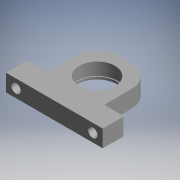
# Autodesk Inventor part: C-BGHKA6902ZZ-30_b_b
Saved by Autodesk Inventor 2017.3 (Build 213256000, 256)
## iProperties
Part Number: C-BGHKA6902ZZ-30_b_b
Material: Generic
Catalog Web Link: www.cadenas.de
Description: C-BGHKA_body-C-VALUE Medium Accuracy Bearings with Housings - T-Shaped
Vendor: MISUMI
Document SubType Name: Modeling
Designer: partserver
Manufacturer: MISUMI
Mass: 19.5015 g
Surface Area: 79.3385 cm^2
Volume: 19.5015 cm^3
Density: 1 g/cm^3
Appearance: PSOLRGB-192-192-192
Category: PARTsolutions
Company: MISUMI
Title: C-BGHKA6902ZZ-30_b
Author: Cadenas PARTsolutions
Comments: C-VALUE Medium Accuracy Bearings with Housings - T-Shaped
PSOL_IDENT_0: {$CADENAS_DATA\23d-libs\misumi\metric\12_bearing_holders\12_cn\c_bghka\c_bghka_body.prj},188 {VTYP=3
PSOL_IDENT_1: D},{NB=C-BGHKA6902ZZ-30_b_b},{LINA=C-BGHKA6902ZZ-30_b},{NN=C-BGHKA_body},{DATE=25.04.2017 02:56:39},
PSOL_IDENT_2: {GEOMDATE=06.02.2013 05:53:00},{VERSION=},{LINEID=60},{WBVAR=HH},{WBNUMERIC=HH}  {NB=C-BGHKA6902ZZ-3
PSOL_IDENT_3: 0_b_b},{LINA=C-BGHKA6902ZZ-30_b},{KT=DUMMY},{PN=C-BGHKA6902ZZ-30},{TYPE=C-BGHKA},{BN=6902ZZ},{HH=30}
PSOL_IDENT_4: ,{HHALG=30,40,50},{DD=15},{H=50},{L1=54},{DD1=6.5},{L=68},{L2=40},{T=12},{S=15},{DDHH=25},{DH7=28},{
PSOL_IDENT_5: B=7},{B11=1.35},{D11=29.4},{R11=16},{R22=1.000},{SRI=28.000},{BN1=6902}
NB: C-BGHKA6902ZZ-30_b_b
NN: C-BGHKA_body
NT: C-VALUE Medium Accuracy Bearings with Housings - T-Shaped
NBSYN: $PN._b_b
LINA: C-BGHKA6902ZZ-30_b
CATALOG: Misumi
PN: C-BGHKA6902ZZ-30
HH: 30
DD: 15
H: 50
L1: 54
DD1: 6.5
L: 68
L2: 40
T: 12
S: 15
DDHH: 25
DH7: 28
B: 7
SUPPLIER: MISUMI
ARTICLENO: C-BGHKA6902ZZ-30_b_b
BOMINFO: C-BGHKA6902ZZ-30_b
CREATOR: CADENAS GmbH
Autodesk Inventor part; units mm, degrees
sketch "Sketch_1" plane through (0, 0, 0) normal (0, 0, 1) x (1, 0, 0)
  line L0 (-34, 14) -> (-34, 0)
  line L1 (-34, 0) -> (34, 0)
  line L2 (34, 0) -> (34, 14)
  arc A0 (34, 14) -> (33, 15) centre (33, 14) ccw
  line L3 (33, 15) -> (21, 15)
  arc A1 (20, 16) -> (21, 15) centre (21, 16) ccw
  line L4 (20, 16) -> (20, 34)
  arc A2 (20, 34) -> (4, 50) centre (4, 34) ccw
  line L5 (4, 50) -> (-4, 50)
  arc A3 (-4, 50) -> (-20, 34) centre (-4, 34) ccw
  line L6 (-20, 34) -> (-20, 16)
  arc A4 (-21, 15) -> (-20, 16) centre (-21, 16) ccw
  line L7 (-21, 15) -> (-33, 15)
  arc A5 (-33, 15) -> (-34, 14) centre (-33, 14) ccw
  constraints: 16 end point, 12 point on circle, 6 centre point
extrude "Extrusion1" add sketch "Sketch_1" along normal mid plane 12
sketch "Sketch_2" plane through (0, 0, 0) normal (1, 0, 0) x (0, 0, -1)
  line L0 (6, 30) -> (-6, 30)
  line L1 (-6, 30) -> (-6, 44)
  line L2 (-6, 44) -> (-4.35, 44)
  line L3 (-4.35, 44) -> (-4.35, 44.7)
  line L4 (-4.35, 44.7) -> (-3, 44.7)
  line L5 (-3, 44.7) -> (-3, 44)
  line L6 (-3, 44) -> (4, 44)
  line L7 (4, 44) -> (4, 42.5)
  line L8 (4, 42.5) -> (6, 42.5)
  line L9 (6, 42.5) -> (6, 30)
  line L10 (6, 30) -> (-6, 30)
  constraints: 22 end point
revolve "Revolution1" cut sketch "Sketch_2" angle 360 about axis through (0, 30, -6) along (0, 0, -1)
sketch "Sketch3" plane through (-34, 0, 6) normal (0, -1, 0) x (1, 0, 0)
  point P0 (61, -6)
hole "Hole1" at (27, 0, 0) direction (0, 1, 0) diameter 6.5 depth 15
pattern_linear "Rectangular Pattern1" count 2 spacing 54 along (-1, 0, 0) of "Hole1"
ref_plane "to_bearing_XY" through (0, 30, -4) normal (0, 0, 1) x (1, 0, 0)
ref_plane "to_bearing_YZ" through (0, 30, -4) normal (1, 0, 0) x (0, 1, 0)
ref_plane "to_bearing_ZX" through (0, 30, -4) normal (0, 1, 0) x (0, 0, 1)
ref_plane "to_snapring_XY" through (0, 30, 4.35) normal (0, 0, 1) x (1, 0, 0)
ref_plane "to_snapring_YZ" through (0, 30, 4.35) normal (1, 0, 0) x (0, 1, 0)
ref_plane "to_snapring_ZX" through (0, 30, 4.35) normal (0, 1, 0) x (0, 0, 1)
body "Solid1"
